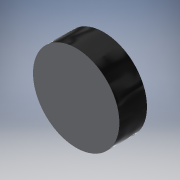
# Autodesk Inventor part: Magnet
Saved by Autodesk Inventor 2019 (Build 230136000, 136)
## iProperties
Created: 2021-10-24
Part Number: Magnet
Material: Generic
Document SubType Name: Modeling
Designer: Mohamed Teleb
Density: 1 g/cm^3
Appearance: Default
Author: Mohamed Teleb
Autodesk Inventor part; units mm, degrees
ref_plane "YZ Plane" through (0, 0, 0) normal (1, 0, 0) x (0, 1, 0)
ref_plane "XZ Plane" through (0, 0, 0) normal (0, 1, 0) x (-1, 0, 0)
ref_plane "XY Plane" through (0, 0, 0) normal (0, 0, 1) x (1, 0, 0)
sketch "Sketch1" plane through (0, 0, 0) normal (0, 0, 1) x (1, 0, 0)
  circle A0 centre (-11.2762, 69.4383) radius 5 projected
  circle A1 centre (-11.2762, 69.4383) radius 5
  point P0 (0, 0)
  constraints: 1 centre point, 1 coincident, 1 concentric
extrude "Extrusion1" add sketch "Sketch1" against normal blind 3.2
body "Solid1"
